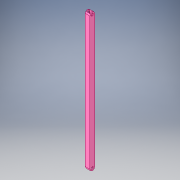
# Autodesk Inventor part: Tie Rod
Saved by Autodesk Inventor 2017 (Build 210142000, 142)
## iProperties
Created: 2017-01-24
Part Number: Tie Rod
Material: Generic
Document SubType Name: Modeling
Designer: Ben
Density: 1 g/cm^3
Appearance: Pink
Author: Ben
Autodesk Inventor part; units mm, degrees
ref_plane "YZ Plane" through (0, 0, 0) normal (1, 0, 0) x (0, 1, 0)
ref_plane "XZ Plane" through (0, 0, 0) normal (0, 1, 0) x (-1, 0, 0)
ref_plane "XY Plane" through (0, 0, 0) normal (0, 0, 1) x (1, 0, 0)
sketch "Sketch1" plane through (0, 0, 0) normal (0, 1, 0) x (-1, 0, 0)
  line L0 (0, 0) -> (12.7, 0)
  line L1 (12.7, 0) -> (12.7, -12.7)
  line L2 (12.7, -12.7) -> (0, -12.7)
  line L3 (0, -12.7) -> (0, 0)
  line L4 (11.1252, -1.5748) -> (1.5748, -1.5748)
  line L5 (1.5748, -1.5748) -> (1.5748, -11.1252)
  line L6 (1.5748, -11.1252) -> (11.1252, -11.1252)
  line L7 (11.1252, -11.1252) -> (11.1252, -1.5748)
  line L8 (6.35, -1.5748) -> (6.35, 0) construction
  line L9 (1.5748, -6.35) -> (0, -6.35) construction
  dimension "d0" = 12.7
  dimension "d1" = 1.5748
  constraints: 20 end point, 5 perpendicular, 4 midpoint, 4 parallel, 2 horizontal, 1 vertical
  measures "d0" distance of L0.start L0.end
  measures "d1" distance between parallel lines of L3 L5
extrude "Extrusion1" add sketch "Sketch1" along normal blind 369.57
sketch "Sketch2" plane through (0, 0, 0) normal (1, 0, 0) x (0, 0, -1)
  line L0 (0, 0) -> (12.7, 0) construction
  line L1 (6.35, 0) -> (6.35, 369.57) construction
  line L2 (0, 369.57) -> (12.7, 369.57) construction
  line L3 (0, 0) -> (0, 369.57) construction
  line L4 (0, 184.785) -> (12.7, 184.785) construction
  circle A0 centre (6.35, 6.35) radius 3.175
  circle A1 centre (6.35, 363.22) radius 3.175
  dimension "d4" = 6.35
  dimension "d5" = 356.87
  constraints: 4 end point, 3 midpoint, 2 centre point, 1 horizontal, 1 point on line, 1 symmetric about line, 1 other
  measures "d4" diameter of A0
  measures "d5" distance of A0.centre A1.centre
extrude "Extrusion2" cut sketch "Sketch2" against normal through all
fillet "Fillet1" radius 6.35 4 edges at (-6.35, 369.57, 0) (-6.35, 369.57, -12.7) (-6.35, 0, 0) (-6.35, 0, -12.7)
body "Solid1"
